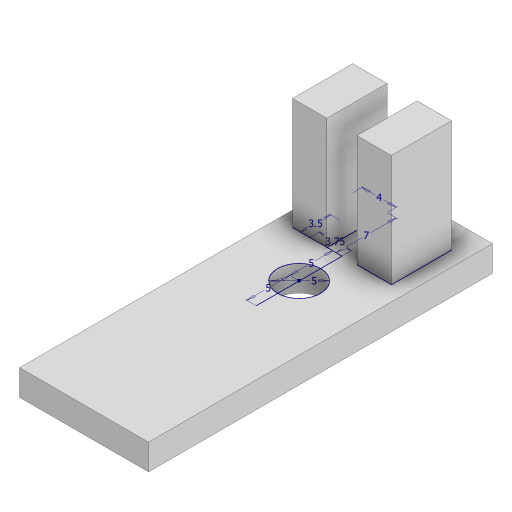
# Autodesk Inventor part: KY 032 INFRERROJO
Saved by Autodesk Inventor 2024 (Build 280153000, 153)
## iProperties
Created: 2024-07-05
Part Number: KY 032 INFRERROJO
Material: Generic
Document SubType Name: Modeling
Designer: Jhuliams
Density: 1 g/cm^3
Appearance: Default
Author: Jhuliams
Autodesk Inventor part; units mm, degrees
ref_plane "YZ Plane" through (0, 0, 0) normal (1, 0, 0) x (0, 1, 0)
ref_plane "XZ Plane" through (0, 0, 0) normal (0, 1, 0) x (-1, 0, 0)
ref_plane "XY Plane" through (0, 0, 0) normal (0, 0, 1) x (1, 0, 0)
sketch "Sketch1" plane through (0, 0, 0) normal (0, 1, 0) x (-1, 0, 0)
  line L0 (7.5, 20) -> (-7.5, 20)
  line L1 (-7.5, 20) -> (-7.5, -20)
  line L2 (-7.5, -20) -> (7.5, -20)
  line L3 (7.5, -20) -> (7.5, 20)
  line L4 (7.5, 20) -> (-7.5, -20) construction
  line L5 (-7.5, 20) -> (7.5, -20) construction
  point P0 (0, 0)
  dimension "d0" = 15
  dimension "d1" = 40
  constraints: 12 end point, 2 midpoint, 2 parallel, 1 horizontal, 1 perpendicular
  measures "d0" distance of L2.end L1.end
  measures "d1" distance of L1.end L0.end
extrude "Extrusion1" add sketch "Sketch1" along normal blind 3
sketch "Sketch2" plane through (0, 3, 0) normal (0, 1, 0) x (1, 0, 0)
  line L0 (0, 0) -> (0, 5)
  circle A0 centre (0, 5) radius 2.5
  line L1 (0, 5) -> (0, 10)
  line L2 (0, 10) -> (-3.75, 10)
  line L3 (-3.75, 10) -> (-3.75, 13.5)
  line L4 (-5.75, 10) -> (-1.75, 10)
  line L5 (-1.75, 10) -> (-1.75, 17)
  line L6 (-1.75, 17) -> (-5.75, 17)
  line L7 (-5.75, 17) -> (-5.75, 10)
  line L8 (-5.75, 10) -> (-1.75, 17) construction
  line L9 (-1.75, 10) -> (-5.75, 17) construction
  line L10 (3.75, 10) -> (3.75, 13.5)
  line L11 (5.75, 10) -> (1.75, 10)
  line L12 (1.75, 10) -> (1.75, 17)
  line L13 (1.75, 17) -> (5.75, 17)
  line L14 (5.75, 17) -> (5.75, 10)
  line L15 (5.75, 10) -> (1.75, 17) construction
  line L16 (1.75, 10) -> (5.75, 17) construction
  dimension "d4" = 5
  dimension "d5" = 5
  dimension "d6" = 5
  dimension "d7" = 3.75
  dimension "d8" = 3.5
  dimension "d9" = 4
  dimension "d10" = 7
  constraints: 34 end point, 6 symmetric about line, 3 vertical, 2 midpoint, 2 parallel, 2 perpendicular, 1 centre point, 1 coincident, 1 horizontal
  measures "d4" distance of L0.start L0.end
  measures "d5" diameter of A0
  measures "d6" distance of L0.end L1.end
  measures "d7" distance of L1.end L2.end
  measures "d8" distance of L2.end L3.end
  measures "d9" distance of L6.end L5.end
  measures "d10" distance of L5.end L4.end
extrude "Extrusion2" add sketch "Sketch2" along normal blind 13 contours L2 L4 L7 L6 L5 | L11 L12 L13 L14
extrude "Extrusion3" cut sketch "Sketch2" against normal blind 13 contours A0 L1 L0 | L0 L1 A0
body "Solid1"
